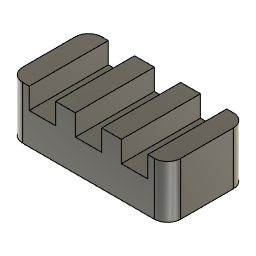
bikeLanePiece (Autodesk Fusion 360 archive; units mm, degrees)
design "bikeLane" references "TactileMapsParameters"
Autodesk Fusion 360 part; units mm, degrees
derive "ExternalDerived1" from "TactileMapsParameters v5"
sketch "Sketch1" plane through (0, 0, 0) normal (0, 0, 1) x (1, 0, 0)
  line L0 (0, 0) -> (12, 0)
  line L1 (12, 0) -> (12, 6)
  line L2 (12, 6) -> (0, 6)
  line L3 (0, 6) -> (0, 0)
  dimension "d18" = 12
  dimension "d19" = 6
  constraint horizontal L0
  constraint vertical L1
  constraint horizontal L2
  constraint vertical L3
  constraint coincident L0.start L3.end
  measures "d18" distance of L0.start L0.end
  measures "d19" distance of L0.start L2.end
extrude "Extrude1" add sketch "Sketch1" along normal blind 0.8
sketch "Sketch2" plane through (0, 0, 0.8) normal (0, 0, 1) x (-1, 0, 0)
  line L0 (0, -6) -> (0, 0)
  line L1 (0, 0) -> (-12, 0)
  line L2 (-12, 0) -> (-12, -6)
  line L3 (-12, -6) -> (0, -6)
  line L4 (0, -6) -> (-1.5, -6)
  line L5 (-1.5, -6) -> (-1.5, 0)
  line L6 (-1.5, 0) -> (0, 0)
  line L7 (0, 0) -> (0, -6)
  line L8 (-3.5, 0) -> (-3.5, -6)
  line L9 (-3.5, -6) -> (-5, -6)
  line L10 (-5, -6) -> (-5, 0)
  line L11 (-5, 0) -> (-3.5, 0)
  line L12 (-7, 0) -> (-7, -6)
  line L13 (-7, -6) -> (-8.5, -6)
  line L14 (-8.5, -6) -> (-8.5, 0)
  line L15 (-8.5, 0) -> (-7, 0)
  line L16 (-10.5, 0) -> (-10.5, -6)
  line L17 (-10.5, -6) -> (-12, -6)
  line L18 (-12, -6) -> (-12, 0)
  line L19 (-12, 0) -> (-10.5, 0)
  dimension "d22" = 1.5
  dimension "d23" = 6
  dimension "d26" = -3.5
  dimension "d27" = 0
  constraint horizontal L4
  constraint vertical L5
  constraint horizontal L6
  constraint vertical L7
  constraint coincident L0.start L3.end
  measures "d22" distance of L0.start L4.end
  measures "d23" distance of L0.start L0.end
extrude "Extrude2" add sketch "Sketch2" along normal blind 3.2 contours L0 L1 L3 L4 L5 L6 L7 | L1 L3 L8 L9 L10 L11 | L1 L3 L12 L13 L14 L15 | L1 L2 L3 L16 L17 L18 L19
extrude "Extrude3" add 3 faces at (2.8333, 2, 0.8) (6.3333, 2, 0.8) (9.8333, 2, 0.8) along direction (0, 0, 1) blind 1.6
fillet "Fillet1" radius 1 4 edges at (12, 0, 2) (0, 0, 2) (12, 6, 2) (0, 6, 2)
equation "length_Ref = 170 mm" comment "Side lengths of base of model"
equation "baseHeight_Ref = 0.4 mm" comment "Height of the base of the model"
equation "sidewalkHeight_Ref = 3.2 mm" comment "Height of sidewalk/walking surface"
equation "sidewalkWidth_Ref = length_Ref / 3" comment "Width of the sidewalk/walking surface"
equation "orientorSize_Ref = 6 mm" comment "Side length of orientation indicator square"
equation "oritentorHeight_Ref = 2.4 mm" comment "Height of the orientation indicator"
equation "braileHeight_Ref = 0.6 mm" comment "Standard height of Braille characters"
equation "filletRadius_Ref = 0.6 mm" comment "Radius of fillets to soften edges"
equation "lineWidth_Ref = 3 mm" comment "Width of crosswalk lines"
equation "lineHeight_Ref = braileHeight_Ref / 2" comment "Height of crosswalk lines"
equation "tabWidth_Ref = length_Ref / 10" comment "Width of tabs to secure adjacent maps together"
equation "tabLength_Ref = length_Ref / 14" comment "Length of tab to secure adjacent maps together"
equation "tabHeight_Ref = sidewalkHeight_Ref / 4" comment "Height of tabs to secure adjacent maps together"
equation "clearance_Ref = 0.4 mm" comment "Clearance around parts that will fit together"
equation "featureHeight_Ref = 1.6 mm" comment "Height of features such as bus stops"
equation "pegSize_Ref = 6 mm" comment "Side length of pegs/holes to connect features to map base"
equation "pegDepth_Ref = sidewalkHeight_Ref / 4" comment "Depth of pegs/holes to connect features to map base"
equation "d18 = 2 * pegSize_Ref"
equation "d19 = pegSize_Ref"
equation "d20 = pegDepth_Ref"
equation "d22 = pegSize_Ref / 4"
equation "d23 = pegSize_Ref"
equation "d28 = 2 * featureHeight_Ref"
equation "d30 = featureHeight_Ref"
